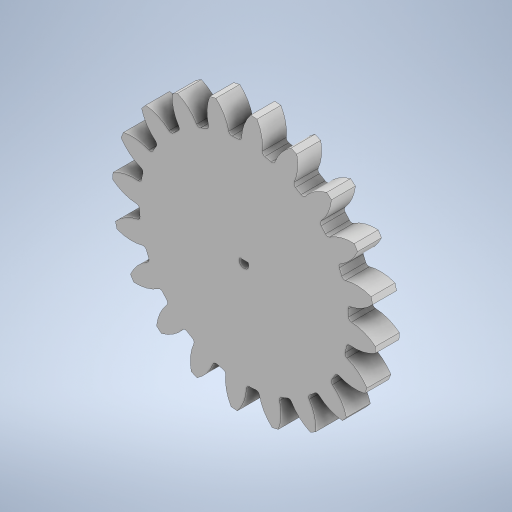
# Autodesk Inventor part: piñon1
Saved by Autodesk Inventor 2023.2 (Build 272271030, 271C)
## iProperties
Created: 2023-03-04
Part Number: piñon1
Material: Generic
Document SubType Name: Modeling
Designer: Cris Pat
Density: 1 g/cm^3
Appearance: Default
Author: Cris Pat
Autodesk Inventor part; units mm, degrees
ref_plane "YZ Plane" through (0, 0, 0) normal (1, 0, 0) x (0, 1, 0)
ref_plane "XZ Plane" through (0, 0, 0) normal (0, 1, 0) x (-1, 0, 0)
ref_plane "XY Plane" through (0, 0, 0) normal (0, 0, 1) x (1, 0, 0)
sketch "Sketch1" plane through (0, 0, 0) normal (0, 0, 1) x (1, 0, 0)
  arc A0 (109.4695, -10.7906) -> (109.8581, -5.5853) centre (0, 0) ccw
  circle A1 centre (0, 0) radius 87.5
  arc A2 (109.8581, -5.5853) -> (87.4759, 2.0527) centre (88.3022, -32.1394) ccw
  arc A3 (86.2012, -15.0201) -> (109.4695, -10.7906) centre (92.0959, 18.6702) ccw
  arc A4 (107.4461, 23.5655) -> (106.2072, 28.6361) centre (0, 0) ccw
  arc A5 (106.2072, 28.6361) -> (82.5602, 28.9837) centre (93.912, -3.2795) ccw
  arc A6 (86.6237, 12.3527) -> (107.4461, 23.5655) centre (81.819, 46.2156) ccw
  arc A7 (94.9052, 55.6148) -> (92.16, 60.0544) centre (0, 0) ccw
  arc A8 (92.16, 60.0544) -> (69.563, 53.0777) centre (90.3291, 25.9014) ccw
  arc A9 (78.5668, 38.5163) -> (94.9052, 55.6148) centre (63.5331, 69.2371) ccw
  arc A10 (73.0743, 82.2201) -> (69.0915, 85.5941) centre (0, 0) ccw
  arc A11 (69.0915, 85.5941) -> (49.7564, 71.976) centre (77.904, 52.5469) ccw
  arc A12 (62.8193, 60.9097) -> (73.0743, 82.2201) centre (39.0281, 85.4812) ccw
  arc A13 (44.0904, 100.7772) -> (39.2599, 102.7553) centre (0, 0) ccw
  arc A14 (39.2599, 102.7553) -> (25.0794, 83.8288) centre (57.8533, 74.0488) ccw
  arc A15 (40.9226, 77.3408) -> (44.0904, 100.7772) centre (10.7028, 93.3578) ccw
  arc A16 (10.7906, 109.4695) -> (5.5853, 109.8581) centre (0, 0) ccw
  arc A17 (5.5853, 109.8581) -> (-2.0527, 87.4759) centre (32.1394, 88.3022) ccw
  arc A18 (15.0201, 86.2012) -> (10.7906, 109.4695) centre (-18.6702, 92.0959) ccw
  arc A19 (-23.5655, 107.4461) -> (-28.6361, 106.2072) centre (0, 0) ccw
  arc A20 (-28.6361, 106.2072) -> (-28.9837, 82.5602) centre (3.2795, 93.912) ccw
  arc A21 (-12.3527, 86.6237) -> (-23.5655, 107.4461) centre (-46.2156, 81.819) ccw
  arc A22 (-55.6148, 94.9052) -> (-60.0544, 92.16) centre (0, 0) ccw
  arc A23 (-60.0544, 92.16) -> (-53.0777, 69.563) centre (-25.9014, 90.3291) ccw
  arc A24 (-38.5163, 78.5668) -> (-55.6148, 94.9052) centre (-69.2371, 63.5331) ccw
  arc A25 (-82.2201, 73.0743) -> (-85.5941, 69.0915) centre (0, 0) ccw
  arc A26 (-85.5941, 69.0915) -> (-71.976, 49.7564) centre (-52.5469, 77.904) ccw
  arc A27 (-60.9097, 62.8193) -> (-82.2201, 73.0743) centre (-85.4812, 39.0281) ccw
  arc A28 (-100.7772, 44.0904) -> (-102.7553, 39.2599) centre (0, 0) ccw
  arc A29 (-102.7553, 39.2599) -> (-83.8288, 25.0794) centre (-74.0488, 57.8533) ccw
  arc A30 (-77.3408, 40.9226) -> (-100.7772, 44.0904) centre (-93.3578, 10.7028) ccw
  arc A31 (-109.4695, 10.7906) -> (-109.8581, 5.5853) centre (0, 0) ccw
  arc A32 (-109.8581, 5.5853) -> (-87.4759, -2.0527) centre (-88.3022, 32.1394) ccw
  arc A33 (-86.2012, 15.0201) -> (-109.4695, 10.7906) centre (-92.0959, -18.6702) ccw
  arc A34 (-107.4461, -23.5655) -> (-106.2072, -28.6361) centre (0, 0) ccw
  arc A35 (-106.2072, -28.6361) -> (-82.5602, -28.9837) centre (-93.912, 3.2795) ccw
  arc A36 (-86.6237, -12.3527) -> (-107.4461, -23.5655) centre (-81.819, -46.2156) ccw
  arc A37 (-94.9052, -55.6148) -> (-92.16, -60.0544) centre (0, 0) ccw
  arc A38 (-92.16, -60.0544) -> (-69.563, -53.0777) centre (-90.3291, -25.9014) ccw
  arc A39 (-78.5668, -38.5163) -> (-94.9052, -55.6148) centre (-63.5331, -69.2371) ccw
  arc A40 (-73.0743, -82.2201) -> (-69.0915, -85.5941) centre (0, 0) ccw
  arc A41 (-69.0915, -85.5941) -> (-49.7564, -71.976) centre (-77.904, -52.5469) ccw
  arc A42 (-62.8193, -60.9097) -> (-73.0743, -82.2201) centre (-39.0281, -85.4812) ccw
  arc A43 (-44.0904, -100.7772) -> (-39.2599, -102.7553) centre (0, 0) ccw
  arc A44 (-39.2599, -102.7553) -> (-25.0794, -83.8288) centre (-57.8533, -74.0488) ccw
  arc A45 (-40.9226, -77.3408) -> (-44.0904, -100.7772) centre (-10.7028, -93.3578) ccw
  arc A46 (-10.7906, -109.4695) -> (-5.5853, -109.8581) centre (0, 0) ccw
  arc A47 (-5.5853, -109.8581) -> (2.0527, -87.4759) centre (-32.1394, -88.3022) ccw
  arc A48 (-15.0201, -86.2012) -> (-10.7906, -109.4695) centre (18.6702, -92.0959) ccw
  arc A49 (23.5655, -107.4461) -> (28.6361, -106.2072) centre (0, 0) ccw
  arc A50 (28.6361, -106.2072) -> (28.9837, -82.5602) centre (-3.2795, -93.912) ccw
  arc A51 (12.3527, -86.6237) -> (23.5655, -107.4461) centre (46.2156, -81.819) ccw
  arc A52 (55.6148, -94.9052) -> (60.0544, -92.16) centre (0, 0) ccw
  arc A53 (60.0544, -92.16) -> (53.0777, -69.563) centre (25.9014, -90.3291) ccw
  arc A54 (38.5163, -78.5668) -> (55.6148, -94.9052) centre (69.2371, -63.5331) ccw
  arc A55 (82.2201, -73.0743) -> (85.5941, -69.0915) centre (0, 0) ccw
  arc A56 (85.5941, -69.0915) -> (71.976, -49.7564) centre (52.5469, -77.904) ccw
  arc A57 (60.9097, -62.8193) -> (82.2201, -73.0743) centre (85.4812, -39.0281) ccw
  arc A58 (100.7772, -44.0904) -> (102.7553, -39.2599) centre (0, 0) ccw
  arc A59 (102.7553, -39.2599) -> (83.8288, -25.0794) centre (74.0488, -57.8533) ccw
  arc A60 (77.3408, -40.9226) -> (100.7772, -44.0904) centre (93.3578, -10.7028) ccw
  arc A61 (-3.4929, 2) -> (3.4929, 2) centre (0, 0) ccw
  line L0 (-3.4929, 2) -> (3.4929, 2)
  point P0 (71.976, -49.7564)
  point P1 (77.3408, -40.9226)
  point P2 (83.8288, -25.0794)
  point P3 (86.6237, 12.3527)
  point P4 (82.5602, 28.9837)
  point P5 (69.563, 53.0777)
  point P6 (62.8193, 60.9097)
  point P7 (49.7564, 71.976)
  point P8 (40.9226, 77.3408)
  point P9 (25.0794, 83.8288)
  point P10 (15.0201, 86.2012)
  point P11 (-2.0527, 87.4759)
  point P12 (-38.5163, 78.5668)
  point P13 (-53.0777, 69.563)
  point P14 (-60.9097, 62.8193)
  point P15 (-71.976, 49.7564)
  point P16 (-77.3408, 40.9226)
  point P17 (-83.8288, 25.0794)
  point P18 (-87.4759, -2.0527)
  point P19 (-78.5668, -38.5163)
  point P20 (-69.563, -53.0777)
  point P21 (-62.8193, -60.9097)
  point P22 (-49.7564, -71.976)
  point P23 (-40.9226, -77.3408)
  point P24 (-25.0794, -83.8288)
  point P25 (-15.0201, -86.2012)
  point P26 (2.0527, -87.4759)
  point P27 (28.9837, -82.5602)
  point P28 (38.5163, -78.5668)
  point P29 (53.0777, -69.563)
  point P30 (60.9097, -62.8193)
  dimension "d10" = 360
  dimension "d19" = 8.05
  dimension "d20" = 2
  constraints: 122 point on circle, 61 centre point, 4 coincident, 2 end point, 1 horizontal, 202 other
  measures "d19" diameter of A61
  measures "d20" distance from line of point (0, 0) L0
extrude "Extrusion1" add sketch "Sketch1" along normal mid plane 20
fillet "Fillet1" radius 2.61 2 edges at (40.9226, 77.3408, 0) (49.7564, 71.976, 0)
pattern_circular "Circular Pattern1" count 20 over 360 about axis through (0, 0, 0) along (0, 0, 1) of "Fillet1"
body "Solid1"
